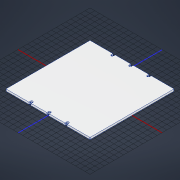
# Autodesk Inventor part: Heatbed
Saved by Autodesk Inventor 2022.2 (Build 262287010, 287A)
## iProperties
Created: 2022-03-13
Part Number: Heatbed
Material: Aluminium 6061
Document SubType Name: Modeling
Designer: sleib
Density: 2.7 g/cm^3
Appearance: Aluminium - flach
Author: sleib
Autodesk Inventor part; units mm, degrees
ref_plane "YZ Plane" through (0, 0, 0) normal (1, 0, 0) x (0, 1, 0)
ref_plane "XZ Plane" through (0, 0, 0) normal (0, 1, 0) x (-1, 0, 0)
ref_plane "XY Plane" through (0, 0, 0) normal (0, 0, 1) x (1, 0, 0)
sketch "Skizze1" plane through (0, 0, 0) normal (0, 1, 0) x (-1, 0, 0)
  line L0 (175, 175) -> (-175, 175)
  line L1 (-175, 175) -> (-175, -175)
  line L2 (-175, -175) -> (175, -175)
  line L3 (175, -175) -> (175, 175)
  line L4 (175, 175) -> (-175, -175) construction
  line L5 (-175, 175) -> (175, -175) construction
  circle A0 centre (75, -168) radius 3.5
  line L6 (78.5, -168) -> (78.5, -175)
  line L7 (71.5, -168) -> (71.5, -175)
  circle A1 centre (-75, -168) radius 3.5
  line L8 (-71.5, -168) -> (-71.5, -175)
  line L9 (-78.5, -168) -> (-78.5, -175)
  circle A2 centre (0, -168) radius 3.5
  line L10 (3.5, -168) -> (3.5, -175)
  line L11 (-3.5, -168) -> (-3.5, -175)
  line L12 (245, 0) -> (-245, 0) construction
  line L13 (0, -245) -> (0, 245) construction
  circle A3 centre (0, -168) radius 5
  line L14 (5, -168) -> (5, -175)
  line L15 (-5, -168) -> (-5, -175)
  line L16 (3.5, -175) -> (-3.5, -175)
  line L17 (-5, -175) -> (5, -175)
  circle A4 centre (75, -168) radius 5
  circle A5 centre (-75, -168) radius 5
  line L18 (80, -168) -> (80, -175)
  line L19 (70, -168) -> (70, -175)
  line L20 (78.5, -175) -> (71.5, -175)
  line L21 (70, -175) -> (80, -175)
  line L22 (-80, -168) -> (-80, -175)
  line L23 (-70, -168) -> (-70, -175)
  line L24 (-70, -175) -> (-80, -175)
  line L25 (-78.5, -175) -> (-71.5, -175)
  circle A6 centre (75, 168) radius 3.5
  line L26 (78.5, 168) -> (78.5, 175)
  line L27 (71.5, 168) -> (71.5, 175)
  circle A7 centre (-75, 168) radius 3.5
  line L28 (-71.5, 168) -> (-71.5, 175)
  line L29 (-78.5, 168) -> (-78.5, 175)
  circle A8 centre (0, 168) radius 3.5
  line L30 (3.5, 168) -> (3.5, 175)
  line L31 (-3.5, 168) -> (-3.5, 175)
  circle A9 centre (0, 168) radius 5
  line L32 (5, 168) -> (5, 175)
  line L33 (-5, 168) -> (-5, 175)
  line L34 (3.5, 175) -> (-3.5, 175)
  line L35 (-5, 175) -> (5, 175)
  circle A10 centre (75, 168) radius 5
  circle A11 centre (-75, 168) radius 5
  line L36 (80, 168) -> (80, 175)
  line L37 (70, 168) -> (70, 175)
  line L38 (78.5, 175) -> (71.5, 175)
  line L39 (70, 175) -> (80, 175)
  line L40 (-80, 168) -> (-80, 175)
  line L41 (-70, 168) -> (-70, 175)
  line L42 (-70, 175) -> (-80, 175)
  line L43 (-78.5, 175) -> (-71.5, 175)
  point P0 (0, 0)
  dimension "d0" = 350
  dimension "d1" = 350
  dimension "d3" = 7
  dimension "d4" = 150
  dimension "d5" = 7
  dimension "d6" = 10
  constraints: 82 end point, 31 symmetric about line, 24 point on circle, 12 centre point, 12 tangent, 12 vertical, 6 coincident, 6 horizontal, 4 equal radius, 2 collinear, 2 horizontal alignment, 2 midpoint, 1 parallel, 1 perpendicular, 1 point on line, 21 other
  measures "d0" distance of L1.end L3.start
  measures "d1" distance of L3.start L0.start
  measures "d3" diameter of A2
  measures "d4" distance of A1.centre A0.centre
  measures "d6" diameter of A3
extrude "Extrusion1" add sketch "Skizze1" against normal blind 8
extrude "Extrusion2" cut sketch "Skizze1" against normal through all contours L26 A10 L27 L0 | L26 A6 L27 A10 | L2 L7 A4 L6 | A6 | A4 L7 A0 L6 | A0 | L30 A9 L31 L0 | L30 A8 L31 A9 | L2 L11 A3 L10 | A8 | A3 L11 A2 L10 | A2 | L28 A11 L29 L0 | L28 A7 L29 A11 | L2 L9 A5 L8 | A7 | A5 L9 A1 L8 | A1 picked at (75.1406, 172.4711) picked at (75.1406, -172.4711) picked at (-0.1406, 172.4711) picked at (0.1406, -172.4711) picked at (-74.8594, 172.4711) picked at (-74.8594, -172.4711)
extrude "Extrusion3" cut sketch "Skizze1" against normal blind 4 contours L36 A10 L26 L0 | A10 L27 A6 L26 | L2 L6 A4 L18 | L27 A10 L37 L0 | A4 L6 A0 L7 | L2 L19 A4 L7 | L32 A9 L30 L0 | A9 L31 A8 L30 | L2 L10 A3 L14 | L31 A9 L33 L0 | A3 L10 A2 L11 | L2 L15 A3 L11 | L41 A11 L28 L0 | A11 L29 A7 L28 | L2 L8 A5 L23 | L29 A11 L40 L0 | A5 L8 A1 L9 | L2 L22 A5 L9 picked at (71.2879, 170.1266) picked at (71.2879, -170.1266) picked at (3.7121, 170.1266) picked at (-3.7121, -170.1266) picked at (-78.7121, 170.1266) picked at (-78.7121, -170.1266)
chamfer "Fase1" distance 1 angle 45 4 edges at (-175, -4, 175) (175, -4, 175) (175, -4, -175) (-175, -4, -175)
